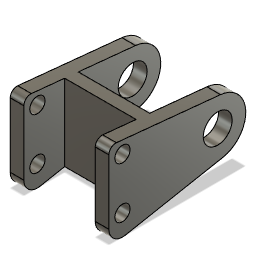
Pedal Connector v1 (Autodesk Fusion 360 design; units mm, degrees)
Autodesk Fusion 360 part; units mm, degrees
sketch "Sketch3" plane through (0, 0, 0) normal (1, 0, 0) x (0, 0, -1)
  circle A0 centre (4, 22) radius 2.25
  circle A1 centre (4, 7) radius 2.25
  line L0 (0, 0) -> (0, 26)
  circle A2 centre (32, 14.5) radius 4.25
  line L1 (12, 24.7968) -> (12, 2.288)
  line L2 (4, 22) -> (4, 7) construction
  line L3 (4, 14.5) -> (32, 14.5) construction
  circle A3 centre (32, 14.5) radius 8.25
  line L4 (0, 26) -> (32.8231, 22.7088)
  line L5 (0, 0) -> (33.5452, 6.396)
  line L6 (16, 24.3957) -> (16, 0.2355)
  dimension "d16" = 4.5
  dimension "d17" = 4.5
  dimension "d18" = 8.5
  dimension "d21" = 4
  dimension "d22" = 4
  dimension "d23" = 15
  dimension "d25" = 4
  dimension "d28" = 8
  dimension "d29" = 7
  dimension "d30" = 90
  dimension "d32" = 4
  dimension "d43" = 4
  dimension "d44" = 16
  constraint coincident L0.start L5.start
  constraint vertical L0
  constraint coincident A0.centre L2.start
  constraint coincident A1.centre L2.end
  constraint midpoint L2 L3.start
  constraint coincident A2.centre L3.end
  constraint parallel L0 L1
  constraint coincident A3 L4.end
  constraint tangent A3 L4
  constraint coincident A3 L5.end
  constraint tangent A3 L5
  constraint coincident L1.start L4
  constraint coincident L1.end L5
  constraint coincident L4 L6.start
  constraint vertical L6
  measures "d16" diameter of A0
  measures "d17" diameter of A1
  measures "d18" diameter of A2
  measures "d21" distance of A1.centre L0
  measures "d22" distance of A0.centre L0
  measures "d23" distance of A0.centre A1.centre
  measures "d25" vertical distance of A0.centre L0.end
  measures "d28" distance of A0.centre L1
  measures "d29" vertical distance of L0.start A1.centre
  measures "d30" angle of L2 L3
  measures "d43" distance of L1 L6
  measures "d44" distance of A2.centre L6
extrude "Extrude2" add sketch "Sketch3" along normal blind 29
fillet "Fillet1" radius 4 1 edges at (14.5, 0, 0)
fillet "Fillet1" radius 2 1 edges at (14.5, 26, 0)
extrude "Extrude3" cut sketch "Sketch3" along normal blind 21 from surface at 4 contours L0 L1 L4 L5 | A3 L4 L5 L6 | A3
equation "d19 = d18 / 2 + 4 mm"
equation "d34 = 21 mm + ( 4 * 2 ) * 1 mm"
equation "d44 = ( 22 / 2 ) * 1 mm + 5 mm"
